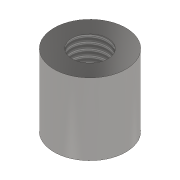
# Autodesk Inventor part: Distanciador para Laterales
Saved by Autodesk Inventor 2020 (Build 240168000, 168)
## iProperties
Created: 2020-07-06
Part Number: Distanciador para Laterales
Material: Steel, High Strength, Low Alloy
Document SubType Name: Modeling
Designer: Pipi
Density: 7.85 g/cm^3
Appearance: Steel - Polished
Author: Pipi
Autodesk Inventor part; units mm, degrees
ref_plane "YZ Plane" through (0, 0, 0) normal (1, 0, 0) x (0, 1, 0)
ref_plane "XZ Plane" through (0, 0, 0) normal (0, 1, 0) x (-1, 0, 0)
ref_plane "XY Plane" through (0, 0, 0) normal (0, 0, 1) x (1, 0, 0)
sketch "Boceto1" plane through (0, 0, 0) normal (0, 1, 0) x (-1, 0, 0)
  circle A0 centre (7.2309, 15.3896) radius 3
  circle A1 centre (7.2309, 15.3896) radius 6
  point P0 (0, 0)
  dimension "d0" = 6
  dimension "d1" = 12
  constraints: 2 centre point, 1 coincident
  measures "d0" diameter of A0
  measures "d1" diameter of A1
extrude "Extrusión1" add sketch "Boceto1" along normal blind 12
thread "Rosca1" size "M6x1" class "6H" standard "ISO Metric profile" length 100
